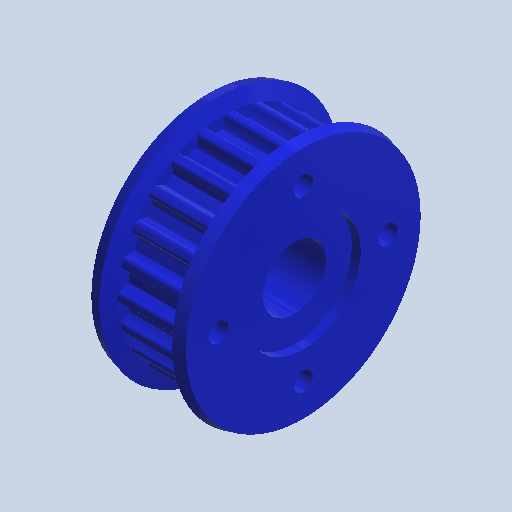
# Autodesk Inventor part: HTPA20S5M100-A-H8_b
Saved by Autodesk Inventor 2024 (Build 280153000, 153)
## iProperties
Category: PARTsolutions
Company: MISUMI
Part Number: HTPA20S5M100-A-H8_b
Material: ABS プラスチック
Catalog Web Link: www.cadenas.de
Description: HTPA__S5M100, HTPA__S5M150, HTPA__S5M250, HTPB__S5M100, HTPB__S5M150, HTPB__S5M250, HTPK__S5M100, HTPK__S5M150, HTPK__S5M250, HTPN__S5M100, HTPN__S5M150, HTPN__S5M250, HTPT__S5M100, HTPT__S5M150, HTPT__S5M250, HTPM__S5M100, HTPM__S5M150, HTPM__S5M250, HTPP__S5M100, HTPP__S5M150, HTPP__S5M250, HTPS__S5M100, HTPS__S5M150_body-High Torque Timing Pulleys S5M Type
Vendor: MISUMI
Document SubType Name: Modeling
Designer: partserver
Manufacturer: MISUMI
Mass: 10.4108 g
Surface Area: 49.6808 cm^2
Volume: 10.4108 cm^3
Density: 1.06 g/cm^3
Appearance: 青 - 壁塗料 - 光沢
PSOL_IDENT_0: {$CADENAS_DATA\23d-libs\misumi\metric\51_timing_pulleys\htpb_s5m\htpb_s5m.prj},732 {VTYP=3D},{NB=HTP
PSOL_IDENT_1: A20S5M100-A-H8_b},{LINA=HTPA20S5M100-A-H8},{NN=HTPA__S5M100, HTPA__S5M150, HTPA__S5M250, HTPB__S5M10
PSOL_IDENT_2: 0, HTPB__S5M150, HTPB__S5M250, HTPK__S5M100, HTPK__S5M150, HTPK__S5M250, HTPN__S5M100, HTPN__S5M150,
PSOL_IDENT_3: HTPN__S5M250, HTPT__S5M100, HTPT__S5M150, HTPT__S5M250, HTPM__S5M100, HTPM__S5M150, HTPM__S5M250, H
PSOL_IDENT_4: TPP__S5M100, HTPP__S5M150, HTPP__S5M250, HTPS__S5M100, HTPS__S5M150_body},{DATE=17.01.2019 01:25:31}
PSOL_IDENT_5: ,{GEOMDATE=28.12.2018 04:09:27},{VERSION=},{LINEID=70},{WBVAR=MATP,ST,TNW,PS,SBS,DD,Z,J,Q,R,S,T,ALT1
PSOL_IDENT_6: ,ALT2,M,QSC,QFC,QTC,ALT3,K,KSC,KFC,KTC,ALT4,ZM,ZSC,ZFC,ZTC,ALT5,ALT6,ALT7,FC,ALT8,SRG,ALT9,BTC,TL,AL
PSOL_IDENT_7: T10,TPC,ALT11,BC,ALT12,SLH},{WBNUMERIC=DD,Z,J,Q,R,S,T,QSC,QFC,QTC,K,KSC,KFC,KTC,ZSC,ZFC,ZTC,FC,SRG,B
PSOL_IDENT_8: TC,TL,BC,SLH}  {NB=HTPA20S5M100-A-H8_b},{LINA=HTPA20S5M100-A-H8},{KT=DUMMY},{PN=HTPA20S5M100-A-H8},{
PSOL_IDENT_9: TYPE=HTPA},{MATP=A2017},{MATPALG= 'A2017','Aluminum Alloy 2000 series','S45C','1045 Carbon Steel Equ
PSOL_IDENT_10: ivalent','SUS304','SUS304' },{ST=CA},{STALG= 'CA','Clear Anodize','BA','Black Anodize','HAT','Hard C
PSOL_IDENT_11: lear Anodize','ENP','Electroless Nickel Plating' },{NT=20},{TNW=S5M100},{TNWALG= 'S5M100','S5M150','
PSOL_IDENT_12: S5M250' },{BW=10},{PS=A},{PSALG= 'A','B' },{SBS=H},{SBSALG= 'H','Round Hole','P','Round Hole + Tap','
PSOL_IDENT_13: N','New JIS Keywayed Bore + Tap (Standard)','NK','New JIS Keywayed Bore + Tap (width 4.0mm, height 1
PSOL_IDENT_14: .8mm)','C','Old JIS Keywayed Bore + Tap','V','Stepped Hole','Y','Both Ends Stepped Hole','WB','Doubl
PSOL_IDENT_15: e Stepped Hole' },{DD=8.00},{DDALG=[6:6/1],6.35,[7:12/1],12.7,[13:20/1]},{DDHA=[6:6/1],6.35,[7:12/1]
PSOL_IDENT_16: ,12.7,[13:20/1]},{DDPA=[6:6/1],6.35,[7:12/1],12.7,[13:16/1]},{DDNA=[8:8/1],[10:16/1]},{DDCA=[10,12,1
PSOL_IDENT_17: 5,16]},{DDVA=[6:6/1],6.35,[7:12/1],12.7,[13:18/1]},{DDY=[6:18/1]},{DDWB=[6:16/1]},{DDHB=},{DDPB=},{D
PSOL_IDENT_18: DNB=},{DDNK=[10:10/1]},{DDCB=},{DDVFB=},{Z=0},{ZALG=[0]},{ZMIN=10.000},{ZAMAX=20.000},{ZBMAX=0.000},
PSOL_IDENT_19: {DDZ=8.000},{J=0.0},{JALG=[0]},{JMIN=2.000},{JMAX=14.000},{JPN=},{Q=0},{QALG=[0]},{QRMIN=10.000},{QR
PSOL_IDENT_20: MAX=20.000},{WBQMIN=12.000},{R=0},{RALG=[0]},{WBRMAX=-2.000},{S=0.0},{SALG=[0]},{SMAX=10.000},{T=0.0
PSOL_IDENT_21: },{TALG=[0]},{TMAX=13.000},{SBSPN=-H8},{A=11},{W=16},{L=0},{PD=31.83},{OD=30.87},{D=0},{DALG=19.000}
PSOL_IDENT_22: ,{DE=24.000},{F=36},{E=24},{TT=1.6},{BBK=0.000},{TTK=0.000},{ALT1=},{ALT1ALG= '','Not applicable' },
PSOL_IDENT_23: {ANG=126.000},{ALT1PN=},{ALT2=},{ALT2ALG= '','w/o Side Tapped Hole','QSC','with QSC (6 Places Side T
PSOL_IDENT_24: apped Hole)','QFC','with QFC (4 Places Side Tapped Hole)','QTC','with QTC (3 Places Side Tapped Hole
PSOL_IDENT_25: )' },{M=N/A},{MALG= 'N/A' },{MFTALG= 'N/A' },{MSALG= 'N/A' },{M3D=0.000},{KDML=0.000},{ML=0.000},{MU
PSOL_IDENT_26: L=0.000},{PITCH=0.000},{QSC=0.0},{QSCALG=0},{QFC=0.0},{QFCALG=0},{QTC=0.0},{QTCALG=0},{QPCDMIN=0.000
PSOL_IDENT_27: },{QPCDMINALG=0.000},{QPCDMAX=20.000},{ALT2PN=},{TAP=0.000},{ALT3=},{ALT3ALG= '','w/o Side Through H
PSOL_IDENT_28: ole','KSC','with KSC (6 Places Side Through Hole)','KFC','with KFC (4 Places Side Through Hole)','KT
PSOL_IDENT_29: C','with KTC (3 Places Side Through Hole)' },{K=0.0},{KALG=0},{KMIN=4.000},{KFTMAX=4.000},{KSMAX=4.0
PSOL_IDENT_30: 00},{KSC=0.0},{KSCALG=0},{KFC=0.0},{KFCALG=0},{KTC=0.0},{KTCALG=0},{KSCMIN=12.000},{KSCMINALG=12},{K
PSOL_IDENT_31: PCDMIN=12.000},{KPCDMINALG=12},{KPCDMAX=20.000},{ALT3PN=},{ALT4=},{ALT4ALG= '','Not applicable' },{A
PSOL_IDENT_32: LT4MIN=18.500},{ALT4MAX=13.500},{ZM=N/A},{ZMALG= 'N/A' },{ZMFTALG= 'N/A' },{ZMSALG= 'N/A' },{ZMDD1=0
PSOL_IDENT_33: .0},{ZMDD2=0.0},{ZMHH=0.0},{ZSC=0.0},{ZSCALG=[0]},{ZFC=0.0},{ZFCALG=[0]},{ZTC=0.0},{ZTCALG=[0]},{ZPC
PSOL_IDENT_34: DMIN=0.000},{ZPCDMINALG=0.000},{ZPCDMAX=20.000},{ALT4PN=},{ALT5=},{ALT5ALG= '','w/o Flange not Attac
PSOL_IDENT_35: hed','NFC','with NFC (Flange not Attached)' },{ALT5PN=},{ALT6=},{ALT6ALG= '','w/o Flange Attached on
PSOL_IDENT_36: One Side Only','RFC','with RFC (Flange Attached on The Boss Side Only)','LFC','with LFC (Flange Att
PSOL_IDENT_37: ached on The Opposite Side Only)' },{ALT6PN=},{ALT7=},{ALT7ALG= '','w/o FC (Flange Cut)','FC','with
PSOL_IDENT_38: FC (Flange Cut)' },{FC=0.0},{FCALG=0},{FCMIN=32.0},{FCMAX=34.0},{ALT7PN=},{ALT8=},{ALT8ALG= '','Not
PSOL_IDENT_39: applicable' },{ALT8ALGALG=20.000},{ALT8DD2=0.000},{ALT8MM=0.000},{ALT8NN=0.000},{QC=0.000},{KC=0.000
PSOL_IDENT_40: },{ZC=0.000},{SRG=0.0},{SRGALG=[0]},{SRGMAX=0.000},{DD2=0.0},{MM=0.00},{NN=0.00},{ALT8PN=},{ALT9=},{
PSOL_IDENT_41: ALT9ALG= '','w/o BTC (Taper for Bearing Holder)','BTC','with BTC (Taper for Bearing Holder)' },{BTC9=
PSOL_IDENT_42: 9.000},{TL9=1.000},{BTC=0},{BTCALG=[0]},{TL=0.0},{TLALG=0},{TLMIN=1.000},{TLMAX=-16.500},{BTCL=0},{B
PSOL_IDENT_43: TCD=0},{ALT9PN=},{WLBCTL=16.000},{ALT10=},{ALT10ALG= '','Not applicable' },{TPC=N/A},{TPCALG= 'N/A'
PSOL_IDENT_44: },{TPCM=4.000},{ALT10PN=},{ALT11=},{ALT11ALG= '','Not applicable' },{BC=0.0},{BCALG=0},{BCMIN=3.000}
PSOL_IDENT_45: ,{BCMAX=-16.500},{M1WBC=8.000},{ALT11PN=},{KTT=11.435},{ALT12=},{ALT12ALG= '','Not applicable' },{SL
PSOL_IDENT_46: H=0},{SLHALG=[0]},{ALT12PN=},{AC=-},{M1=4.000},{M1L=3.000}
NB: HTPA20S5M100-A-H8_b
NN: 0
NT: 20
NBSYN: $PN._b
LINA: HTPA20S5M100-A-H8
CATALOG: Misumi
PN: HTPA20S5M100-A-H8
MATP: Aluminum Alloy 2000 series
ST: Clear Anodize
TNW: S5M100
BW: 10
PS: A
SBS: Round Hole
DD: 8
Z: 0
J: 0
Q: 0
R: 0
S: 0
T: 0
A: 11
W: 16
L: 0
PD: 31.83
OD: 30.87
D: 0
F: 36
E: 24
TT: 1.6
ALT1: Not applicable
ALT2: w/o Side Tapped Hole
M: N/A
QSC: 0
QFC: 0
QTC: 0
ALT3: w/o Side Through Hole
K: 0
KSC: 0
KFC: 0
KTC: 0
ALT4: Not applicable
ZM: N/A
ZMDD1: 0
ZMDD2: 0
ZMHH: 0
ZSC: 0
ZFC: 0
ZTC: 0
ALT5: w/o Flange not Attached
ALT6: w/o Flange Attached on One Side Only
ALT7: w/o FC (Flange Cut)
FC: 0
ALT8: Not applicable
SRG: 0
DD2: 0
MM: 0
ALT9: w/o BTC (Taper for Bearing Holder)
BTC: 0
TL: 0
BTCL: 0
BTCD: 0
ALT10: Not applicable
TPC: N/A
ALT11: Not applicable
BC: 0
ALT12: Not applicable
SLH: 0
AC: -
SUPPLIER: MISUMI
ARTICLENO: HTPA20S5M100-A-H8_b
BOMINFO: HTPA20S5M100-A-H8
CREATOR: CADENAS GmbH
Title: HTPA20S5M100-A-H8
Author: Cadenas PARTsolutions
Comments: High Torque Timing Pulleys S5M Type
Autodesk Inventor part; units mm, degrees
note: some values were not read from the file. Chosen so that the rebuilt part matches the saved one: pattern direction of "Circular Pattern1".
ref_plane "YZ Plane" through (0, 0, 0) normal (1, 0, 0) x (0, 1, 0)
ref_plane "XZ Plane" through (0, 0, 0) normal (0, 1, 0) x (-1, 0, 0)
ref_plane "XY Plane" through (0, 0, 0) normal (0, 0, 1) x (1, 0, 0)
sketch "_____2" plane through (0, 0, 0) normal (0, 0, 1) x (1, 0, 0)
  line L0 (0, 0) -> (0, 17.3)
  line L1 (0, 17.3) -> (0.9, 17.3)
  line L2 (0.9, 17.3) -> (0.9, 17.6122)
  line L3 (0.9, 17.6122) -> (0.2846, 19.9087)
  line L4 (0.2846, 19.9087) -> (1.8301, 20.3228)
  line L5 (1.8301, 20.3228) -> (2.5, 17.8228)
  line L6 (2.5, 17.8228) -> (13.5, 17.8228)
  line L7 (13.5, 17.8228) -> (14.1699, 20.3228)
  line L8 (14.1699, 20.3228) -> (15.7154, 19.9087)
  line L9 (15.7154, 19.9087) -> (15.1, 17.6122)
  line L10 (15.1, 17.6122) -> (15.1, 17.3)
  line L11 (15.1, 17.3) -> (16, 17.3)
  line L12 (16, 17.3) -> (16, 0)
  line L13 (16, 0) -> (0, 0)
  line L14 (8, 17.8228) -> (8, 0) construction
  line L15 (0, 17.3) -> (0, 19.8324)
  line L16 (0, 19.8324) -> (0.2846, 19.9087)
  line L17 (16, 17.3) -> (16, 19.8324)
  line L18 (16, 19.8324) -> (15.7154, 19.9087)
  line L19 (13.5, 17.8228) -> (13.5, 0)
  line L20 (2.5, 17.8228) -> (2.5, 0)
  point P0 (0.344, 17.3)
  point P1 (15.656, 17.3)
  dimension "d40" = 17.8228
  dimension "d41" = 16
  dimension "d42" = 11
  dimension "d43" = 105
  dimension "d53" = 1.6
  dimension "d54" = 17.3
  dimension "d55" = 0.9
  dimension "d56" = 2.5
  constraints: 42 end point, 10 perpendicular, 3 vertical, 2 collinear, 2 midpoint, 2 point on line, 1 coincident, 1 horizontal, 1 parallel, 1 vertical alignment, 5 other
  measures "d40" distance between parallel lines of L13 L6
  measures "d41" distance of L12.end L0.start
  measures "d42" distance of L5.end L6.end
  measures "d43" angle of L6 L5
  measures "d53" distance of L3.end L4.end
  measures "d54" distance of L0.start L0.end
  measures "d55" distance of L0.end L1.end
  measures "d56" vertical distance of L5.end L4.end
revolve "Revolution1" add sketch "_____2" angle 360 about axis through (16, 0, 0) along (1, 0, 0)
sketch "Sketch2" plane through (0, 0, 0) normal (1, 0, 0) x (0, 0, -1)
  point P0 (0, 0)
  point P1 (0, 0)
  constraints: 1 coincident
hole "軸穴" at (0, 0, 0) direction (1, 0, 0) diameter 10.6 end through all
sketch "_____6" plane through (2.5, 0, 0) normal (1, 0, 0) x (0, 0, -1)
  arc A0 (-1.517, 17.3066) -> (-2.1097, 17.6975) centre (-2.0446, 17.1514) ccw
  arc A1 (-1.517, 17.3066) -> (-0.8856, 16.1275) centre (1.625, 18.2305) ccw
  arc A2 (-0.8856, 16.1275) -> (-0.6833, 16.0383) centre (-0.6939, 16.288) ccw
  arc A3 (0.6833, 16.0383) -> (-0.6833, 16.0383) centre (0, 0) ccw
  arc A4 (0.6833, 16.0383) -> (0.8856, 16.1275) centre (0.6939, 16.288) ccw
  arc A5 (0.8856, 16.1275) -> (1.517, 17.3066) centre (-1.625, 18.2305) ccw
  arc A6 (2.1097, 17.6975) -> (1.517, 17.3066) centre (2.0446, 17.1514) ccw
  line L0 (2.1097, 17.6975) -> (2.1097, 18.1808)
  arc A7 (2.1097, 18.1808) -> (-2.1097, 18.1808) centre (0, 0) ccw
  line L1 (-2.1097, 18.1808) -> (-2.1097, 17.6975)
  line L2 (0, 0) -> (0, 18.3028)
  arc A8 (2.1097, 17.6975) -> (-2.1097, 17.6975) centre (0, 0) ccw construction
  dimension "d44" = 0.55
  dimension "d45" = 3.275
  dimension "d46" = 0.25
  dimension "d47" = 2.25
  dimension "d49" = 18.3028
  dimension "d50" = 0.48
  dimension "d52" = 3.25
  constraints: 20 point on circle, 9 centre point, 7 tangent, 6 end point, 3 coincident, 3 equal radius, 2 vertical, 4 other
  measures "d44" radius of A6
  measures "d45" radius of A5
  measures "d46" radius of A4
  measures "d47" radial gap between concentric circles of A7 A3
  measures "d49" distance of L2.start L2.end
  measures "d50" radial gap between concentric circles of A7 A8
  measures "d52" distance of A1.centre A5.centre
extrude "Extrusion1" cut sketch "_____6" along normal blind 11
pattern_circular "Circular Pattern1" count 23 over 360 about axis through (8, 0, 0) along (1, 0, 0) of "Extrusion1"
sketch "スケッチ10" plane through (0, 0, 0) normal (1, 0, 0) x (0, 0, -1)
  point P0 (0, 0)
  point P1 (0, 14.3)
  point P2 (0, -14.3)
  point P3 (-14.3, 0)
  point P4 (0, -14.3)
  point P5 (14.3, 0)
  dimension "d59" = 360
  dimension "d61" = 14.3
  dimension "d117" = 360
  constraints: 1 vertical alignment, 8 other
  measures "d61" distance of point (0, 0) point (0, 14.3)
hole "セットカラー取付穴" at (0, 14.3, 0) at (0, -14.3, 0) at (0, 0, -14.3) at (0, 0, 14.3) direction (1, 0, 0) diameter 3.2 end through all
sketch "スケッチ11" plane through (0, 0, 0) normal (1, 0, 0) x (0, 1, 0)
  circle A0 centre (0, 0) radius 17.3
  circle A1 centre (0, 0) radius 5.3
  dimension "d69" = 34.6
  dimension "d70" = 10.6
  constraints: 2 centre point, 2 coincident
  measures "d69" diameter of A0
  measures "d70" diameter of A1
extrude "ボス" [suppressed]
sketch "スケッチ12" plane through (-10, 0, 0) normal (-1, 0, 0) x (0, 0, 1)
  circle A0 centre (0, 0) radius 11 projected
  line L0 (-3.2787, 10.5) -> (3.2787, 10.5)
  dimension "d73" = 16.8
  constraints: 2 end point, 2 point on circle, 1 horizontal
extrude "押し出し7" [suppressed]
sketch "スケッチ13" plane through (-10, 10.5, 3.2787) normal (0, 1, 0) x (1, 0, 0)
  line L0 (0, 0) -> (0, 6.5574) projected
  point P0 (10, 3.2787)
  point P1 (5, 3.2787)
  point P2 (0, 3.2787)
  dimension "d76" = 5
  constraints: 1 horizontal alignment, 1 midpoint
  measures "d76" distance from line of L0 point (5, 3.279)
hole "イモネジ穴" [suppressed]
sketch "スケッチ14" plane through (-5, 5.7, 0) normal (0, 1, 0) x (1, 0, 0)
  line L0 (2.4, 0) -> (1.2, -2.0785)
  line L1 (1.2, -2.0785) -> (-1.2, -2.0785)
  line L2 (-1.2, -2.0785) -> (-2.4, 0)
  line L3 (-2.4, 0) -> (-1.2, 2.0785)
  line L4 (-1.2, 2.0785) -> (1.2, 2.0785)
  line L5 (1.2, 2.0785) -> (2.4, 0)
  circle A0 centre (0, 0) radius 2.4
  point P0 (1.2, -2.0785)
  point P1 (1.2, -2.0785)
  point P2 (1.2, 2.0785)
  point P3 (1.2, 2.0785)
  point P4 (-1.2, 2.0785)
  point P5 (-1.2, 2.0785)
  point P6 (-2.4, 0)
  point P7 (-2.4, 0)
  point P8 (-1.2, -2.0785)
  dimension "d84" = 4.8
  constraints: 12 end point, 2 coincident, 1 horizontal, 14 other
  measures "d84" distance of L0.start L2.end
extrude "インサートナット" [suppressed]
sketch "スケッチ15" plane through (-5, 5.7, 0) normal (0, -1, 0) x (0, 0, -1)
  point P0 (0, 0)
hole "穴6" [suppressed]
chamfer "面取り1" [suppressed]
chamfer "面取り2" [suppressed]
sketch "スケッチ16" plane through (16, 0, 0) normal (1, 0, 0) x (0, 0, -1)
  line L0 (11.2567, 8.3872) -> (11.2567, -8.3872) construction
  line L1 (11.2567, -8.3872) -> (16.4081, -8.3872) construction
  line L2 (16.4081, -8.3872) -> (16.4081, 8.3872) construction
  line L3 (16.4081, 8.3872) -> (11.2567, 8.3872) construction
  circle A0 centre (0, 0) radius 19.8324 projected
  point P0 (0, 0)
  point P1 (13.1432, 14.852)
  point P2 (13.8324, -8.3872)
  point P3 (16.4081, 0)
  dimension "歯数" = 23
  dimension "d108" = 19.8324
  dimension "d109" = 13.8324
  constraints: 2 midpoint, 1 horizontal alignment, 1 vertical alignment, 4 other
  measures "d108" distance of point (13.143, 14.852) point (0, 0)
  measures "d109" horizontal distance of point (13.832, -8.387) point (0, 0)
extrude "押し出し9" [suppressed]
sketch "スケッチ17" plane through (0, 0, 0) normal (-1, 0, 0) x (0, 0, 1)
  circle A0 centre (0, 0) radius 9.7
  dimension "d112" = 19.4
  constraints: 1 centre point, 1 coincident
  measures "d112" diameter of A0
extrude "押し出し10" cut sketch "スケッチ17" against normal blind 1.5
equation "\"d42\" = 歯幅"
equation "\"d1\" = 穴径"
equation "\"d49\" = 0.795775 * 歯数"
equation "\"d8\" = 歯幅"
equation "\"d61\" = 0.5 * 穴間隔"
equation "\"d69\" = 2 * d54"
equation "\"d70\" = d1"
equation "\"d76\" = 0.5 * d71"
equation "\"d74\" = d71"
equation "\"d82\" = 0.5 * d69"
equation "\"d84\" = d101"
equation "\"d97\" = -0.5 * d103 + 0.5 * d104"
equation "\"d100\" = -0.5 * d103 + 0.5 * d104"
equation "\"歯数\" = 23"
equation "\"歯幅\" = 11"
equation "\"穴径\" = 10.6"
equation "\"d71\" = 10"
equation "\"d101\" = 4.8"
equation "\"d103\" = 2.458734"
equation "\"d104\" = 3"
equation "\"穴間隔\" = 28.6"
body "Solid1"
